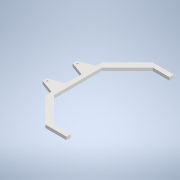
# Autodesk Inventor part: Arm
Saved by Autodesk Inventor 2020 (Build 240168000, 168)
## iProperties
Created: 2020-02-26
Part Number: Arm
Material: Generic
Document SubType Name: Modeling
Designer: shrey
Density: 1 g/cm^3
Appearance: Default
Author: shrey
Autodesk Inventor part; units mm, degrees
ref_plane "YZ Plane" through (0, 0, 0) normal (1, 0, 0) x (0, 1, 0)
ref_plane "XZ Plane" through (0, 0, 0) normal (0, 1, 0) x (-1, 0, 0)
ref_plane "XY Plane" through (0, 0, 0) normal (0, 0, 1) x (1, 0, 0)
sketch "Sketch1" plane through (0, 0, 0) normal (0, 1, 0) x (-1, 0, 0)
  line L0 (4.6355, 50.8) -> (-4.6355, 50.8)
  line L1 (-4.6355, 50.8) -> (-4.6355, -50.8)
  line L2 (-4.6355, -50.8) -> (4.6355, -50.8)
  line L3 (4.6355, -50.8) -> (4.6355, 50.8)
  line L4 (4.6355, 50.8) -> (-4.6355, -50.8) construction
  line L5 (-4.6355, 50.8) -> (4.6355, -50.8) construction
  line L6 (4.6355, 50.8) -> (4.6355, 75.7051) construction
  line L7 (4.6355, -50.8) -> (4.6355, -91.0918) construction
  line L8 (-4.6355, 50.8) -> (4.6355, 60.071)
  line L9 (4.6355, 60.071) -> (-49.246, 113.9525)
  line L10 (-49.246, 113.9525) -> (-58.517, 104.6815)
  line L11 (-58.517, 104.6815) -> (-4.6355, 50.8)
  line L12 (-4.6355, 50.8) -> (8.4757, 50.8) construction
  line L13 (-4.6355, -50.8) -> (4.6355, -60.071)
  line L14 (4.6355, -60.071) -> (-49.246, -113.9525)
  line L15 (-49.246, -113.9525) -> (-58.517, -104.6815)
  line L16 (-58.517, -104.6815) -> (-4.6355, -50.8)
  line L17 (-4.6355, -50.8) -> (8.4757, -50.8) construction
  line L18 (4.6355, 60.071) -> (4.6355, 50.8)
  line L19 (4.6355, -50.8) -> (4.6355, -60.071)
  line L20 (4.6355, 50.8) -> (4.6355, 38.1)
  line L21 (4.6355, 41.021) -> (4.6355, 60.071)
  line L22 (4.6355, 31.75) -> (4.6355, 41.021)
  line L23 (48.5075, 0) -> (-17.0034, 0) construction
  line L24 (-58.517, -104.6815) -> (-58.517, 104.6815) construction
  line L25 (-49.246, -113.9525) -> (-58.517, -113.9525)
  line L26 (-58.517, -113.9525) -> (-58.517, -104.6815)
  line L27 (-58.517, -104.6815) -> (-94.077, -104.6815)
  line L28 (-94.077, -104.6815) -> (-94.077, -113.9525)
  line L29 (-94.077, -113.9525) -> (-58.517, -113.9525)
  line L30 (-58.517, 104.6815) -> (-94.077, 104.6815)
  line L31 (-94.077, 104.6815) -> (-94.077, 113.9525)
  line L32 (-94.077, 113.9525) -> (-49.246, 113.9525)
  line L33 (55.1879, -32) -> (4.6355, -32) construction
  line L34 (4.6355, -32) -> (4.6355, -60.071)
  line L35 (4.6355, 22.7291) -> (4.6355, 50.8)
  line L36 (33.8455, 32) -> (4.6355, 32) construction
  line L37 (4.6355, 32) -> (4.6355, 60.071)
  line L38 (4.6355, 27.3645) -> (33.8455, 27.3645) construction
  line L39 (33.8455, 27.3645) -> (33.8455, 36.6355)
  line L40 (33.8455, 36.6355) -> (4.6355, 36.6355) construction
  line L41 (4.6355, 36.6355) -> (4.6355, 27.3645)
  line L42 (4.6355, 27.3645) -> (33.8455, 36.6355) construction
  line L43 (33.8455, 27.3645) -> (4.6355, 36.6355) construction
  line L44 (4.6355, -32) -> (33.8455, -32) construction
  line L45 (4.6355, -36.6355) -> (33.8455, -36.6355) construction
  line L46 (33.8455, -36.6355) -> (33.8455, -27.3645)
  line L47 (33.8455, -27.3645) -> (4.6355, -27.3645) construction
  line L48 (4.6355, -27.3645) -> (4.6355, -36.6355)
  line L49 (4.6355, -36.6355) -> (33.8455, -27.3645) construction
  line L50 (33.8455, -36.6355) -> (4.6355, -27.3645) construction
  line L51 (33.8455, -32) -> (28.7655, -32) construction
  circle A0 centre (28.7655, -32) radius 1.85
  line L52 (33.8455, 32) -> (28.7655, 32) construction
  circle A1 centre (28.7655, 32) radius 1.85
  line L53 (33.8455, -36.6355) -> (4.6355, -47.2671)
  line L54 (33.8455, -36.6355) -> (64.9301, -36.6355) construction
  line L55 (33.8455, -27.3645) -> (4.6355, -16.7329)
  line L56 (33.8455, -27.3645) -> (64.9301, -27.3645) construction
  line L57 (33.8455, 27.3645) -> (4.6355, 16.7329)
  line L58 (33.8455, 27.3645) -> (64.9301, 27.3645) construction
  line L59 (33.8455, 36.6355) -> (4.6355, 47.2671)
  line L60 (33.8455, 36.6355) -> (64.9301, 36.6355) construction
  point P0 (0, 0)
  point P1 (33.8455, 45.6585)
  point P2 (33.8455, 45.6585)
  point P3 (33.8455, 45.6585)
  dimension "d0" = 9.271
  dimension "d1" = 101.6
  dimension "d2" = 45
  dimension "d3" = 76.2
  dimension "d4" = 45
  dimension "d5" = 76.2
  dimension "d8" = 12.7
  dimension "d12" = 35.56
  dimension "d17" = 35.56
  dimension "d28" = 9.271
  dimension "d29" = 50.5524
  dimension "d30" = 29.21
  dimension "d31" = 9.271
  dimension "d32" = 5.08
  dimension "d33" = 3.7
  dimension "d34" = 5.08
  dimension "d35" = 3.7
  dimension "d36" = 160
  dimension "d37" = 160
  dimension "d38" = 160
  dimension "d39" = 160
  constraints: 122 end point, 12 parallel, 11 horizontal, 10 point on line, 7 perpendicular, 6 equal length, 4 vertical, 2 centre point, 2 coincident, 2 collinear, 2 midpoint
  measures "d0" distance of L2.end L1.end
  measures "d1" distance of L1.end L0.end
  measures "d2" angle of L12 L8
  measures "d3" distance of L9.end L8.end
  measures "d4" angle of L13 L17
  measures "d5" distance of L13.end L14.end
  measures "d8" distance of L20.start L20.end
  measures "d12" distance of L27.end L15.end
  measures "d17" distance of L10.end L30.end
  measures "d28" distance of L39.end L38.end
  measures "d29" distance of L33.start L33.end
  measures "d30" distance of L33.end L44.end
  measures "d31" distance of L46.end L45.end
  measures "d32" distance of L44.end L51.end
  measures "d33" diameter of A0
  measures "d34" distance of L36.start L52.end
  measures "d35" diameter of A1
  measures "d36" angle of L53 L54
  measures "d37" angle of L56 L55
  measures "d38" angle of L57 L58
  measures "d39" angle of L60 L59
extrude "Extrusion4" add sketch "Sketch1" along normal blind 6.35
fillet "Fillet4" radius 3.175 6 edges at (49.246, 3.175, 113.9525) (49.246, 3.175, -113.9525) (-4.6355, 3.175, -47.2671) (-4.6355, 3.175, 16.7329) (-4.6355, 3.175, 47.2671) (-4.6355, 3.175, -16.7329)
fillet "Fillet5" radius 3.175 4 edges at (-33.8455, 3.175, 36.6355) (-33.8455, 3.175, -27.3645) (-33.8455, 3.175, 27.3645) (-33.8455, 3.175, -36.6355)
fillet "Fillet6" radius 3.175 2 edges at (4.6355, 3.175, 50.8) (4.6355, 3.175, -50.8)
body "Solid4"
